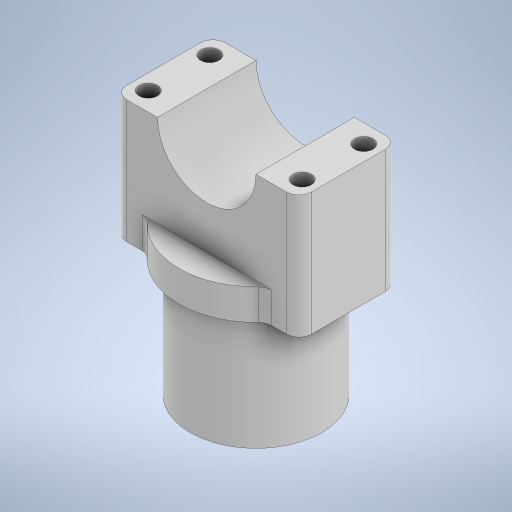
# Autodesk Inventor part: base1
Saved by Autodesk Inventor 2023 (Build 270158000, 158)
## iProperties
Created: 2022-11-13
Part Number: base1
Material: Generic
Document SubType Name: Modeling
Designer: andre
Density: 1 g/cm^3
Appearance: Default
Author: andre
Autodesk Inventor part; units mm, degrees
ref_plane "YZ Plane" through (0, 0, 0) normal (1, 0, 0) x (0, 1, 0)
ref_plane "XZ Plane" through (0, 0, 0) normal (0, 1, 0) x (-1, 0, 0)
ref_plane "XY Plane" through (0, 0, 0) normal (0, 0, 1) x (1, 0, 0)
sketch "Sketch1" plane through (0, 0, 0) normal (0, 1, 0) x (-1, 0, 0)
  circle A0 centre (0, 0) radius 10.7
  dimension "d0" = 21.4
  constraints: 1 centre point, 1 coincident
  measures "d0" diameter of A0
extrude "Extrusion1" add sketch "Sketch1" along normal blind 19
sketch "Sketch2" plane through (0, 19, 0) normal (0, 1, 0) x (1, 0, 0)
  circle A0 centre (0, 0) radius 12.5
  circle A1 centre (0, 0) radius 10.7 projected
  line L0 (-15, 8) -> (15, 8)
  line L1 (15, 8) -> (15, -8)
  line L2 (15, -8) -> (-15, -8)
  line L3 (-15, -8) -> (-15, 8)
  line L4 (0, 0) -> (1.899, 0)
  line L5 (0, 0) -> (0, 1.5989)
  point P0 (-12.5, 0)
  point P1 (9.6047, -8)
  point P2 (-9.6047, 8)
  point P3 (12.5, 0)
  point P4 (-9.6047, -8)
  point P5 (9.6047, 8)
  dimension "d9" = 25
  dimension "d10" = 21.4
  dimension "d14" = 30
  dimension "d15" = 16
  constraints: 12 end point, 2 horizontal, 2 parallel, 1 centre point, 1 coincident, 1 perpendicular, 1 vertical, 2 other
  measures "d9" diameter of A0
  measures "d10" diameter of A1
  measures "d14" distance of L0.start L0.end
  measures "d15" distance of L2.end L0.start
extrude "Extrusion2" add sketch "Sketch2" along normal blind 5
sketch "Sketch3" plane through (0, 0, 0) normal (0, 0, 1) x (1, 0, 0)
  line L0 (10.7, 0) -> (-10.7, 0) projected
  line L1 (9.6047, 19) -> (15, 19) projected
  line L2 (15, 19) -> (15, 24) projected
  line L3 (-15, 24) -> (-9.6047, 24) projected
  line L4 (-15, 19) -> (-15, 24) projected
  circle A0 centre (0, 39) radius 15
  circle A1 centre (0, 39) radius 8
  line L5 (-15, 19) -> (-15, 24) projected
  line L6 (-15, 39) -> (-15, 24)
  line L7 (15, 39) -> (15, 24)
  line L8 (-15, 39) -> (15, 39)
  line L9 (9.6047, 24) -> (15, 24) projected
  line L10 (9.6047, 19) -> (9.6047, 24) projected
  line L11 (-15, 19) -> (-9.6047, 19) projected
  line L12 (-9.6047, 19) -> (-9.6047, 24) projected
  line L13 (-15, 24) -> (15, 24)
  point P0 (0, 0)
  point P1 (-8, 19)
  point P2 (8, 19)
  point P3 (10.7, 19)
  point P4 (-10.7, 19)
  point P5 (8, 39)
  point P6 (-8, 39)
  dimension "d16" = 30
  dimension "d17" = 30
  dimension "d18" = 16
  constraints: 8 end point, 2 centre point, 2 collinear, 2 point on circle, 1 coincident, 1 perpendicular, 1 tangent, 1 vertical
  measures "d16" distance of L3.start L2.end
  measures "d17" diameter of A0
  measures "d18" diameter of A1
extrude "Extrusion3" add sketch "Sketch3" along normal mid plane 16 contours L13 A0 L7 L9 | L13 L3 L6 A0 | A0 L8 A1 picked at (-12.5413, 37.8874)
sketch "Sketch4" plane through (0, 19, 0) normal (0, -1, 0) x (1, 0, 0)
  arc A0 (-9.6047, -8) -> (9.6047, -8) centre (0, 0) ccw projected
  line L0 (15, -8) -> (9.6047, -8) projected
  line L1 (15, 8) -> (15, -8) projected
  line L2 (9.6047, 8) -> (15, 8) projected
  arc A1 (9.6047, 8) -> (-9.6047, 8) centre (0, 0) ccw projected
  line L3 (-15, 8) -> (-9.6047, 8) projected
  line L4 (-15, -8) -> (-15, 8) projected
  line L5 (-9.6047, -8) -> (-15, -8) projected
  circle A2 centre (0, 0) radius 10.7 projected
  line L6 (12.5, 5) -> (-12.5, 5)
  line L7 (-12.5, 5) -> (-12.5, -5)
  line L8 (-12.5, -5) -> (12.5, -5)
  line L9 (12.5, -5) -> (12.5, 5)
  line L10 (0, 0) -> (0, 1.5128)
  line L11 (0, 0) -> (1.2888, 0)
  dimension "d19" = 10
  dimension "d20" = 25
  constraints: 12 end point, 4 coincident, 2 horizontal, 2 parallel, 1 perpendicular, 1 point on line, 1 vertical, 2 other
  measures "d19" distance of L8.end L6.start
  measures "d20" distance of L7.end L8.end
hole "Hole1" at (12.5, 19, 5) at (12.5, 19, -5) at (-12.5, 19, -5) at (-12.5, 19, 5) direction (0, 1, 0) diameter 3 end through all
fillet "Fillet1" radius 2 8 edges at (-15, 29, 8) (15, 29, 8) (15, 29, -8) (-15, 29, -8) (9.6047, 21.5, 8) (-9.6047, 21.5, 8) (9.6047, 21.5, -8) (-9.6047, 21.5, -8)
equation "\"d17\" = d16"
body "Solid1"
